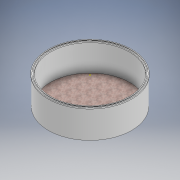
# Autodesk Inventor part: ObservatoryFloor
Saved by Autodesk Inventor 2022 (Build 260153000, 153)
## iProperties
Created: 2021-04-25
Part Number: ObservatoryFloor
Material: Generic
Document SubType Name: Modeling
Designer: Mick Veldhuis
Density: 1 g/cm^3
Appearance: Default
Author: Mick Veldhuis
Autodesk Inventor part; units mm, degrees
ref_plane "YZ Plane" through (0, 0, 0) normal (1, 0, 0) x (0, 1, 0)
ref_plane "XZ Plane" through (0, 0, 0) normal (0, 1, 0) x (-1, 0, 0)
ref_plane "XY Plane" through (0, 0, 0) normal (0, 0, 1) x (1, 0, 0)
sketch "Sketch1" plane through (0, 0, 0) normal (0, 1, 0) x (-1, 0, 0)
  circle A0 centre (0, 0) radius 2500
  constraints: 1 centre point, 1 coincident
extrude "Floor" add sketch "Sketch1" along normal blind 50
sketch "Sketch2" plane through (0, 50, 0) normal (0, 1, 0) x (1, 0, 0)
  circle A0 centre (0, 0) radius 2400
  circle A1 centre (0, 0) radius 2500
  constraints: 2 centre point, 2 coincident
extrude "Wall" add sketch "Sketch2" along normal blind 1600
sketch "Sketch3" plane through (0, 1650, 0) normal (0, 1, 0) x (1, 0, 0)
  point P0 (0, 0)
sketch "Sketch4" plane through (0, 1650, 0) normal (0, 1, 0) x (1, 0, 0)
  circle A0 centre (0, 0) radius 2525
  circle A1 centre (0, 0) radius 2375
  dimension "d4" = 5050
  dimension "d5" = 4750
  constraints: 2 centre point, 2 coincident
  measures "d4" diameter of A0
  measures "d5" diameter of A1
extrude "Extrusion3" add sketch "Sketch4" along normal blind 50
sketch "Sketch5" plane through (0, 1700, 0) normal (0, 1, 0) x (1, 0, 0)
  circle A0 centre (0, 0) radius 2525
  circle A1 centre (0, 0) radius 2375 projected
  circle A2 centre (0, 0) radius 2375
  circle A3 centre (0, 0) radius 2425
  circle A4 centre (0, 0) radius 2475
  constraints: 4 centre point, 3 coincident
extrude "Extrusion4" add sketch "Sketch5" along normal blind 20
body "Solid1"
